Autodesk Inventor part; units mm, degrees
(part 2 of 2)
  arc A137 (24.76, -34.525) -> (24.36, -34.125) centre (24.36, -34.525) ccw
  line L182 (132.16, -34.125) -> (135.12, -34.125)
  arc A138 (135.52, -34.525) -> (135.12, -34.125) centre (135.12, -34.525) ccw
  line L183 (135.52, -34.525) -> (135.52, -47.125)
  arc A139 (132.380606, -52.964154) -> (135.52, -47.125) centre (128.52, -47.125) ccw
  arc A140 (131.76, -52.630488) -> (132.380606, -52.964154) centre (132.16, -52.630488) ccw
  line L184 (131.76, -52.630488) -> (131.76, -34.525)
  arc A141 (132.16, -34.125) -> (131.76, -34.525) centre (132.16, -34.525) ccw
  line L185 (120.76, -34.525) -> (120.76, -53.725)
  arc A142 (120.36, -54.125) -> (120.76, -53.725) centre (120.36, -53.725) ccw
  line L186 (120.36, -54.125) -> (116.16, -54.125)
  arc A143 (115.76, -53.725) -> (116.16, -54.125) centre (116.16, -53.725) ccw
  line L187 (115.76, -53.725) -> (115.76, -34.525)
  arc A144 (116.16, -34.125) -> (115.76, -34.525) centre (116.16, -34.525) ccw
  line L188 (116.16, -34.125) -> (120.36, -34.125)
  arc A145 (120.76, -34.525) -> (120.36, -34.125) centre (120.36, -34.525) ccw
  line L189 (120.36, 2) -> (117.866824, 2)
  arc A146 (117.866824, 2) -> (115.76, 14.782046) centre (65.9053, 0) ccw
  line L190 (115.76, 14.782046) -> (115.76, 29.725)
  arc A147 (116.16, 30.125) -> (115.76, 29.725) centre (116.16, 29.725) ccw
  line L191 (116.16, 30.125) -> (120.36, 30.125)
  arc A148 (120.76, 29.725) -> (120.36, 30.125) centre (120.36, 29.725) ccw
  line L192 (120.76, 29.725) -> (120.76, 2.4)
  arc A149 (120.36, 2) -> (120.76, 2.4) centre (120.36, 2.4) ccw
  line L193 (13.943776, 2) -> (12.16, 2)
  arc A150 (11.76, 2.4) -> (12.16, 2) centre (12.16, 2.4) ccw
  line L194 (11.76, 2.4) -> (11.76, 29.725)
  arc A151 (12.16, 30.125) -> (11.76, 29.725) centre (12.16, 29.725) ccw
  line L195 (12.16, 30.125) -> (16.36, 30.125)
  arc A152 (16.76, 29.725) -> (16.36, 30.125) centre (16.36, 29.725) ccw
  line L196 (16.76, 29.725) -> (16.76, 16.992336)
  arc A153 (16.76, 16.992336) -> (13.943776, 2) centre (65.9053, 0) ccw
  line L197 (135.12, 2) -> (132.16, 2)
  arc A154 (131.76, 2.4) -> (132.16, 2) centre (132.16, 2.4) ccw
  line L198 (131.76, 2.4) -> (131.76, 29.725)
  arc A155 (132.16, 30.125) -> (131.76, 29.725) centre (132.16, 29.725) ccw
  line L199 (132.16, 30.125) -> (135.12, 30.125)
  arc A156 (135.52, 29.725) -> (135.12, 30.125) centre (135.12, 29.725) ccw
  line L200 (135.52, 29.725) -> (135.52, 2.4)
  arc A157 (135.12, 2) -> (135.52, 2.4) centre (135.12, 2.4) ccw
  line L201 (124.16, -2) -> (128.36, -2)
  arc A158 (128.76, -2.4) -> (128.36, -2) centre (128.36, -2.4) ccw
  line L202 (128.76, -2.4) -> (128.76, -29.725)
  arc A159 (128.36, -30.125) -> (128.76, -29.725) centre (128.36, -29.725) ccw
  line L203 (128.36, -30.125) -> (124.16, -30.125)
  arc A160 (123.76, -29.725) -> (124.16, -30.125) centre (124.16, -29.725) ccw
  line L204 (123.76, -29.725) -> (123.76, -2.4)
  arc A161 (124.16, -2) -> (123.76, -2.4) centre (124.16, -2.4) ccw
  line L205 (8.36, 2) -> (5.4, 2)
  arc A162 (5, 2.4) -> (5.4, 2) centre (5.4, 2.4) ccw
  line L206 (5, 2.4) -> (5, 29.725)
  arc A163 (5.4, 30.125) -> (5, 29.725) centre (5.4, 29.725) ccw
  line L207 (5.4, 30.125) -> (8.36, 30.125)
  arc A164 (8.76, 29.725) -> (8.36, 30.125) centre (8.36, 29.725) ccw
  line L208 (8.76, 29.725) -> (8.76, 2.4)
  arc A165 (8.36, 2) -> (8.76, 2.4) centre (8.36, 2.4) ccw
  line L209 (120.76, -2.4) -> (120.76, -29.725)
  arc A166 (120.36, -30.125) -> (120.76, -29.725) centre (120.36, -29.725) ccw
  line L210 (120.36, -30.125) -> (116.16, -30.125)
  arc A167 (115.76, -29.725) -> (116.16, -30.125) centre (116.16, -29.725) ccw
  line L211 (115.76, -29.725) -> (115.76, -14.782046)
  arc A168 (115.76, -14.782046) -> (117.866824, -2) centre (65.9053, 0) ccw
  line L212 (117.866824, -2) -> (120.36, -2)
  arc A169 (120.76, -2.4) -> (120.36, -2) centre (120.36, -2.4) ccw
  line L213 (123.76, 2.4) -> (123.76, 29.725)
  arc A170 (124.16, 30.125) -> (123.76, 29.725) centre (124.16, 29.725) ccw
  line L214 (124.16, 30.125) -> (128.36, 30.125)
  arc A171 (128.76, 29.725) -> (128.36, 30.125) centre (128.36, 29.725) ccw
  line L215 (128.76, 29.725) -> (128.76, 2.4)
  arc A172 (128.36, 2) -> (128.76, 2.4) centre (128.36, 2.4) ccw
  line L216 (128.36, 2) -> (124.16, 2)
  arc A173 (123.76, 2.4) -> (124.16, 2) centre (124.16, 2.4) ccw
  line L217 (135.52, -2.4) -> (135.52, -29.725)
  arc A174 (135.12, -30.125) -> (135.52, -29.725) centre (135.12, -29.725) ccw
  line L218 (135.12, -30.125) -> (132.16, -30.125)
  arc A175 (131.76, -29.725) -> (132.16, -30.125) centre (132.16, -29.725) ccw
  line L219 (131.76, -29.725) -> (131.76, -2.4)
  arc A176 (132.16, -2) -> (131.76, -2.4) centre (132.16, -2.4) ccw
  line L220 (132.16, -2) -> (135.12, -2)
  arc A177 (135.52, -2.4) -> (135.12, -2) centre (135.12, -2.4) ccw
  line L221 (8.76, -2.4) -> (8.76, -29.725)
  arc A178 (8.36, -30.125) -> (8.76, -29.725) centre (8.36, -29.725) ccw
  line L222 (8.36, -30.125) -> (5.4, -30.125)
  arc A179 (5, -29.725) -> (5.4, -30.125) centre (5.4, -29.725) ccw
  line L223 (5, -29.725) -> (5, -2.4)
  arc A180 (5.4, -2) -> (5, -2.4) centre (5.4, -2.4) ccw
  line L224 (5.4, -2) -> (8.36, -2)
  arc A181 (8.76, -2.4) -> (8.36, -2) centre (8.36, -2.4) ccw
  arc A182 (13.943776, -2) -> (16.76, -16.992336) centre (65.9053, 0) ccw
  line L225 (16.76, -16.992336) -> (16.76, -29.725)
  arc A183 (16.36, -30.125) -> (16.76, -29.725) centre (16.36, -29.725) ccw
  line L226 (16.36, -30.125) -> (12.16, -30.125)
  arc A184 (11.76, -29.725) -> (12.16, -30.125) centre (12.16, -29.725) ccw
  line L227 (11.76, -29.725) -> (11.76, -2.4)
  arc A185 (12.16, -2) -> (11.76, -2.4) centre (12.16, -2.4) ccw
  line L228 (12.16, -2) -> (13.943776, -2)
  arc A186 (8.170583, -52.982797) -> (12.16, -54.125) centre (13.033749, -43.53513) ccw
  line L229 (12.16, -34.125) -> (8.36, -34.125)
  line L230 (143.52, -61.875) -> (143.52, 62.125)
  line L231 (143.52, 62.125) -> (-2.75, 62.125)
  point P0 (0, 0)
  point P1 (8.183841, -52.989609)
  point P2 (12.091903, -54.119161)
  constraints: 3 point on circle, 2 end point, 1 centre point, 1 point on line
extrude "Extrusion11" cut sketch "Sketch13" against normal through all contours L17 L229 A34 L33 A33 A186 A17 A18 L19 A19
sketch "Sketch14" plane through (0, 0, 16.5) normal (0, 0, 1) x (1, 0, 0)
  arc A0 (13.943776, -2) -> (16.76, -16.992336) centre (65.9053, 0) ccw
  line L0 (16.76, -16.992336) -> (16.76, -29.725)
  arc A1 (16.36, -30.125) -> (16.76, -29.725) centre (16.36, -29.725) ccw
  line L1 (16.36, -30.125) -> (12.16, -30.125)
  arc A2 (11.76, -29.725) -> (12.16, -30.125) centre (12.16, -29.725) ccw
  line L2 (11.76, -29.725) -> (11.76, -2.4)
  arc A3 (12.16, -2) -> (11.76, -2.4) centre (12.16, -2.4) ccw
  line L3 (12.16, -2) -> (13.943776, -2)
  line L4 (8.76, -2.4) -> (8.76, -29.725)
  arc A4 (8.36, -30.125) -> (8.76, -29.725) centre (8.36, -29.725) ccw
  line L5 (8.36, -30.125) -> (5.4, -30.125)
  arc A5 (5, -29.725) -> (5.4, -30.125) centre (5.4, -29.725) ccw
  line L6 (5, -29.725) -> (5, -2.4)
  arc A6 (5.4, -2) -> (5, -2.4) centre (5.4, -2.4) ccw
  line L7 (5.4, -2) -> (8.36, -2)
  arc A7 (8.76, -2.4) -> (8.36, -2) centre (8.36, -2.4) ccw
  line L8 (135.52, -2.4) -> (135.52, -29.725)
  arc A8 (135.12, -30.125) -> (135.52, -29.725) centre (135.12, -29.725) ccw
  line L9 (135.12, -30.125) -> (132.16, -30.125)
  arc A9 (131.76, -29.725) -> (132.16, -30.125) centre (132.16, -29.725) ccw
  line L10 (131.76, -29.725) -> (131.76, -2.4)
  arc A10 (132.16, -2) -> (131.76, -2.4) centre (132.16, -2.4) ccw
  line L11 (132.16, -2) -> (135.12, -2)
  arc A11 (135.52, -2.4) -> (135.12, -2) centre (135.12, -2.4) ccw
  line L12 (123.76, 2.4) -> (123.76, 29.725)
  arc A12 (124.16, 30.125) -> (123.76, 29.725) centre (124.16, 29.725) ccw
  line L13 (124.16, 30.125) -> (128.36, 30.125)
  arc A13 (128.76, 29.725) -> (128.36, 30.125) centre (128.36, 29.725) ccw
  line L14 (128.76, 29.725) -> (128.76, 2.4)
  arc A14 (128.36, 2) -> (128.76, 2.4) centre (128.36, 2.4) ccw
  line L15 (128.36, 2) -> (124.16, 2)
  arc A15 (123.76, 2.4) -> (124.16, 2) centre (124.16, 2.4) ccw
  line L16 (120.76, -2.4) -> (120.76, -29.725)
  arc A16 (120.36, -30.125) -> (120.76, -29.725) centre (120.36, -29.725) ccw
  line L17 (120.36, -30.125) -> (116.16, -30.125)
  arc A17 (115.76, -29.725) -> (116.16, -30.125) centre (116.16, -29.725) ccw
  line L18 (115.76, -29.725) -> (115.76, -14.782046)
  arc A18 (115.76, -14.782046) -> (117.866824, -2) centre (65.9053, 0) ccw
  line L19 (117.866824, -2) -> (120.36, -2)
  arc A19 (120.76, -2.4) -> (120.36, -2) centre (120.36, -2.4) ccw
  line L20 (8.36, 2) -> (5.4, 2)
  arc A20 (5, 2.4) -> (5.4, 2) centre (5.4, 2.4) ccw
  line L21 (5, 2.4) -> (5, 29.725)
  arc A21 (5.4, 30.125) -> (5, 29.725) centre (5.4, 29.725) ccw
  line L22 (5.4, 30.125) -> (8.36, 30.125)
  arc A22 (8.76, 29.725) -> (8.36, 30.125) centre (8.36, 29.725) ccw
  line L23 (8.76, 29.725) -> (8.76, 2.4)
  arc A23 (8.36, 2) -> (8.76, 2.4) centre (8.36, 2.4) ccw
  line L24 (124.16, -2) -> (128.36, -2)
  arc A24 (128.76, -2.4) -> (128.36, -2) centre (128.36, -2.4) ccw
  line L25 (128.76, -2.4) -> (128.76, -29.725)
  arc A25 (128.36, -30.125) -> (128.76, -29.725) centre (128.36, -29.725) ccw
  line L26 (128.36, -30.125) -> (124.16, -30.125)
  arc A26 (123.76, -29.725) -> (124.16, -30.125) centre (124.16, -29.725) ccw
  line L27 (123.76, -29.725) -> (123.76, -2.4)
  arc A27 (124.16, -2) -> (123.76, -2.4) centre (124.16, -2.4) ccw
  line L28 (135.12, 2) -> (132.16, 2)
  arc A28 (131.76, 2.4) -> (132.16, 2) centre (132.16, 2.4) ccw
  line L29 (131.76, 2.4) -> (131.76, 29.725)
  arc A29 (132.16, 30.125) -> (131.76, 29.725) centre (132.16, 29.725) ccw
  line L30 (132.16, 30.125) -> (135.12, 30.125)
  arc A30 (135.52, 29.725) -> (135.12, 30.125) centre (135.12, 29.725) ccw
  line L31 (135.52, 29.725) -> (135.52, 2.4)
  arc A31 (135.12, 2) -> (135.52, 2.4) centre (135.12, 2.4) ccw
  line L32 (13.943776, 2) -> (12.16, 2)
  arc A32 (11.76, 2.4) -> (12.16, 2) centre (12.16, 2.4) ccw
  line L33 (11.76, 2.4) -> (11.76, 29.725)
  arc A33 (12.16, 30.125) -> (11.76, 29.725) centre (12.16, 29.725) ccw
  line L34 (12.16, 30.125) -> (16.36, 30.125)
  arc A34 (16.76, 29.725) -> (16.36, 30.125) centre (16.36, 29.725) ccw
  line L35 (16.76, 29.725) -> (16.76, 16.992336)
  arc A35 (16.76, 16.992336) -> (13.943776, 2) centre (65.9053, 0) ccw
  line L36 (120.36, 2) -> (117.866824, 2)
  arc A36 (117.866824, 2) -> (115.76, 14.782046) centre (65.9053, 0) ccw
  line L37 (115.76, 14.782046) -> (115.76, 29.725)
  arc A37 (116.16, 30.125) -> (115.76, 29.725) centre (116.16, 29.725) ccw
  line L38 (116.16, 30.125) -> (120.36, 30.125)
  arc A38 (120.76, 29.725) -> (120.36, 30.125) centre (120.36, 29.725) ccw
  line L39 (120.76, 29.725) -> (120.76, 2.4)
  arc A39 (120.36, 2) -> (120.76, 2.4) centre (120.36, 2.4) ccw
  line L40 (120.76, -34.525) -> (120.76, -53.725)
  arc A40 (120.36, -54.125) -> (120.76, -53.725) centre (120.36, -53.725) ccw
  line L41 (120.36, -54.125) -> (116.16, -54.125)
  arc A41 (115.76, -53.725) -> (116.16, -54.125) centre (116.16, -53.725) ccw
  line L42 (115.76, -53.725) -> (115.76, -34.525)
  arc A42 (116.16, -34.125) -> (115.76, -34.525) centre (116.16, -34.525) ccw
  line L43 (116.16, -34.125) -> (120.36, -34.125)
  arc A43 (120.76, -34.525) -> (120.36, -34.125) centre (120.36, -34.525) ccw
  line L44 (132.16, -34.125) -> (135.12, -34.125)
  arc A44 (135.52, -34.525) -> (135.12, -34.125) centre (135.12, -34.525) ccw
  line L45 (135.52, -34.525) -> (135.52, -47.125)
  arc A45 (132.380606, -52.964154) -> (135.52, -47.125) centre (128.52, -47.125) ccw
  arc A46 (131.76, -52.630488) -> (132.380606, -52.964154) centre (132.16, -52.630488) ccw
  line L46 (131.76, -52.630488) -> (131.76, -34.525)
  arc A47 (132.16, -34.125) -> (131.76, -34.525) centre (132.16, -34.525) ccw
  line L47 (24.76, -34.525) -> (24.76, -53.725)
  arc A48 (24.36, -54.125) -> (24.76, -53.725) centre (24.36, -53.725) ccw
  line L48 (24.36, -54.125) -> (20.16, -54.125)
  arc A49 (19.76, -53.725) -> (20.16, -54.125) centre (20.16, -53.725) ccw
  line L49 (19.76, -53.725) -> (19.76, -34.525)
  arc A50 (20.16, -34.125) -> (19.76, -34.525) centre (20.16, -34.525) ccw
  line L50 (20.16, -34.125) -> (24.36, -34.125)
  arc A51 (24.76, -34.525) -> (24.36, -34.125) centre (24.36, -34.525) ccw
  arc A52 (23.520345, 30.125) -> (19.76, 23.971051) centre (65.9053, 0) ccw
  line L51 (19.76, 23.971051) -> (19.76, 29.725)
  arc A53 (20.16, 30.125) -> (19.76, 29.725) centre (20.16, 29.725) ccw
  line L52 (20.16, 30.125) -> (23.520345, 30.125)
  line L53 (107.76, 34.525) -> (107.76, 53.725)
  arc A54 (108.16, 54.125) -> (107.76, 53.725) centre (108.16, 53.725) ccw
  line L54 (108.16, 54.125) -> (112.36, 54.125)
  arc A55 (112.76, 53.725) -> (112.36, 54.125) centre (112.36, 53.725) ccw
  line L55 (112.76, 53.725) -> (112.76, 34.525)
  arc A56 (112.36, 34.125) -> (112.76, 34.525) centre (112.36, 34.525) ccw
  line L56 (112.36, 34.125) -> (108.16, 34.125)
  arc A57 (107.76, 34.525) -> (108.16, 34.125) centre (108.16, 34.525) ccw
  arc A58 (108.290254, -30.125) -> (112.76, -22.552984) centre (65.9053, 0) ccw
  line L57 (112.76, -22.552984) -> (112.76, -29.725)
  arc A59 (112.36, -30.125) -> (112.76, -29.725) centre (112.36, -29.725) ccw
  line L58 (112.36, -30.125) -> (108.290254, -30.125)
  line L59 (128.76, -34.525) -> (128.76, -53.725)
  arc A60 (128.36, -54.125) -> (128.76, -53.725) centre (128.36, -53.725) ccw
  line L60 (128.36, -54.125) -> (124.16, -54.125)
  arc A61 (123.76, -53.725) -> (124.16, -54.125) centre (124.16, -53.725) ccw
  line L61 (123.76, -53.725) -> (123.76, -34.525)
  arc A62 (124.16, -34.125) -> (123.76, -34.525) centre (124.16, -34.525) ccw
  line L62 (124.16, -34.125) -> (128.36, -34.125)
  arc A63 (128.76, -34.525) -> (128.36, -34.125) centre (128.36, -34.525) ccw
  line L63 (16.36, 34.125) -> (12.16, 34.125)
  arc A64 (11.76, 34.525) -> (12.16, 34.125) centre (12.16, 34.525) ccw
  line L64 (11.76, 34.525) -> (11.76, 53.725)
  arc A65 (12.16, 54.125) -> (11.76, 53.725) centre (12.16, 53.725) ccw
  line L65 (12.16, 54.125) -> (16.36, 54.125)
  arc A66 (16.76, 53.725) -> (16.36, 54.125) centre (16.36, 53.725) ccw
  line L66 (16.76, 53.725) -> (16.76, 34.525)
  arc A67 (16.36, 34.125) -> (16.76, 34.525) centre (16.36, 34.525) ccw
  line L67 (8.36, 34.125) -> (5.4, 34.125)
  arc A68 (5, 34.525) -> (5.4, 34.125) centre (5.4, 34.525) ccw
  line L68 (5, 34.525) -> (5, 47.125)
  arc A69 (8.139394, 52.964154) -> (5, 47.125) centre (12, 47.125) ccw
  arc A70 (8.76, 52.630488) -> (8.139394, 52.964154) centre (8.36, 52.630488) ccw
  line L69 (8.76, 52.630488) -> (8.76, 34.525)
  arc A71 (8.36, 34.125) -> (8.76, 34.525) centre (8.36, 34.525) ccw
  line L70 (115.76, 34.525) -> (115.76, 53.725)
  arc A72 (116.16, 54.125) -> (115.76, 53.725) centre (116.16, 53.725) ccw
  line L71 (116.16, 54.125) -> (120.36, 54.125)
  arc A73 (120.76, 53.725) -> (120.36, 54.125) centre (120.36, 53.725) ccw
  line L72 (120.76, 53.725) -> (120.76, 34.525)
  arc A74 (120.36, 34.125) -> (120.76, 34.525) centre (120.36, 34.525) ccw
  line L73 (120.36, 34.125) -> (116.16, 34.125)
  arc A75 (115.76, 34.525) -> (116.16, 34.125) centre (116.16, 34.525) ccw
  line L74 (83.76, -12.185449) -> (83.76, 0.332706)
  line L75 (83.76, 0.332706) -> (88.76, 13.193084)
  line L76 (88.76, 13.193084) -> (88.76, -9.998135)
  line L77 (88.76, -9.998135) -> (83.76, -12.185449)
  line L78 (80.76, -21.138342) -> (80.76, -42.477499)
  arc A76 (75.76, -43.907686) -> (80.76, -42.477499) centre (65.9053, 0) ccw
  line L79 (75.76, -43.907686) -> (75.76, -23.325656)
  line L80 (75.76, -23.325656) -> (80.76, -21.138342)
  line L81 (91.76, -8.685747) -> (91.76, 20.90931)
  line L82 (91.76, 20.90931) -> (96.47099, 33.026332)
  arc A77 (96.76, 32.756488) -> (96.47099, 33.026332) centre (65.9053, 0) ccw
  line L83 (96.76, 32.756488) -> (96.76, -6.498433)
  line L84 (96.76, -6.498433) -> (91.76, -8.685747)
  line L85 (107.76, -1.686342) -> (107.76, 16.528281)
  arc A78 (110.904226, -0.31086) -> (107.76, 16.528281) centre (65.9053, 0) ccw
  line L86 (110.904226, -0.31086) -> (107.76, -1.686342)
  line L87 (104.76, -10.639235) -> (104.76, -22.700491)
  arc A79 (99.76, -29.645561) -> (104.76, -22.700491) centre (65.9053, 0) ccw
  line L88 (99.76, -29.645561) -> (99.76, -12.826549)
  line L89 (99.76, -12.826549) -> (104.76, -10.639235)
  line L90 (75.76, -0.926469) -> (75.76, 24.326911)
  line L91 (75.76, 24.326911) -> (80.76, 20.268157)
  line L92 (80.76, 20.268157) -> (80.76, 11.933908)
  line L93 (80.76, 11.933908) -> (75.76, -0.926469)
  line L94 (72.76, -27.960124) -> (72.76, -44.474859)
  arc A80 (67.76, -44.961763) -> (72.76, -44.474859) centre (65.9053, 0) ccw
  line L95 (67.76, -44.961763) -> (67.76, -40.820501)
  line L96 (67.76, -40.820501) -> (72.76, -27.960124)
  line L97 (24.76, 34.125) -> (20.16, 34.125)
  arc A81 (19.76, 34.525) -> (20.16, 34.125) centre (20.16, 34.525) ccw
  line L98 (19.76, 34.525) -> (19.76, 53.725)
  arc A82 (20.16, 54.125) -> (19.76, 53.725) centre (20.16, 53.725) ccw
  line L99 (20.16, 54.125) -> (24.36, 54.125)
  arc A83 (24.76, 53.725) -> (24.36, 54.125) centre (24.36, 53.725) ccw
  line L100 (24.76, 53.725) -> (24.76, 34.125)
  line L101 (51.76, -42.718971) -> (51.76, 42.718971)
  arc A84 (52.72419, 43.026252) -> (51.76, 42.718971) centre (65.9053, 0) ccw
  line L102 (52.72419, 43.026252) -> (56.76, 39.750179)
  line L103 (56.76, 39.750179) -> (56.76, -44.060907)
  arc A85 (51.76, -42.718971) -> (56.76, -44.060907) centre (65.9053, 0) ccw
  line L104 (48.76, -49.092145) -> (48.76, -53.725)
  arc A86 (48.36, -54.125) -> (48.76, -53.725) centre (48.36, -53.725) ccw
  line L105 (48.36, -54.125) -> (44.16, -54.125)
  arc A87 (43.76, -53.725) -> (44.16, -54.125) centre (44.16, -53.725) ccw
  line L106 (43.76, -53.725) -> (43.76, -47.048759)
  arc A88 (43.76, -47.048759) -> (48.76, -49.092145) centre (65.9053, 0) ccw
  line L107 (51.76, 50.03909) -> (51.76, 53.725)
  arc A89 (52.16, 54.125) -> (51.76, 53.725) centre (52.16, 53.725) ccw
  line L108 (52.16, 54.125) -> (56.36, 54.125)
  arc A90 (56.76, 53.725) -> (56.36, 54.125) centre (56.36, 53.725) ccw
  line L109 (56.76, 53.725) -> (56.76, 51.189486)
  arc A91 (56.76, 51.189486) -> (51.76, 50.03909) centre (65.9053, 0) ccw
  arc A92 (43.76, -39.173788) -> (48.76, -41.605753) centre (65.9053, 0) ccw
  line L110 (43.76, -39.173788) -> (43.76, 39.173788)
  arc A93 (48.76, 41.605753) -> (43.76, 39.173788) centre (65.9053, 0) ccw
  line L111 (48.76, 41.605753) -> (48.76, -41.605753)
  line L112 (108.16, -34.125) -> (112.36, -34.125)
  arc A94 (112.76, -34.525) -> (112.36, -34.125) centre (112.36, -34.525) ccw
  line L113 (112.76, -34.525) -> (112.76, -53.725)
  arc A95 (112.36, -54.125) -> (112.76, -53.725) centre (112.36, -53.725) ccw
  line L114 (112.36, -54.125) -> (108.16, -54.125)
  arc A96 (107.76, -53.725) -> (108.16, -54.125) centre (108.16, -53.725) ccw
  line L115 (107.76, -53.725) -> (107.76, -34.525)
  arc A97 (108.16, -34.125) -> (107.76, -34.525) centre (108.16, -34.525) ccw
  line L116 (59.76, -42.079676) -> (59.76, 37.314927)
  line L117 (59.76, 37.314927) -> (64.76, 33.256172)
  line L118 (64.76, 33.256172) -> (64.76, -29.219299)
  line L119 (64.76, -29.219299) -> (59.76, -42.079676)
  line L120 (23.520345, -30.125) -> (20.16, -30.125)
  arc A98 (19.76, -29.725) -> (20.16, -30.125) centre (20.16, -29.725) ccw
  line L121 (19.76, -29.725) -> (19.76, -23.971051)
  arc A99 (19.76, -23.971051) -> (23.520345, -30.125) centre (65.9053, 0) ccw
  line L122 (27.76, -23.873334) -> (27.76, 23.873334)
  arc A100 (32.76, 30.436641) -> (27.76, 23.873334) centre (65.9053, 0) ccw
  line L123 (32.76, 30.436641) -> (32.76, -30.436641)
  arc A101 (27.76, -23.873334) -> (32.76, -30.436641) centre (65.9053, 0) ccw
  line L124 (27.76, 35.34029) -> (27.76, 53.725)
  arc A102 (28.16, 54.125) -> (27.76, 53.725) centre (28.16, 53.725) ccw
  line L125 (28.16, 54.125) -> (32.36, 54.125)
  arc A103 (32.76, 53.725) -> (32.36, 54.125) centre (32.36, 53.725) ccw
  line L126 (32.76, 53.725) -> (32.76, 40.067307)
  arc A104 (32.76, 40.067307) -> (27.76, 35.34029) centre (65.9053, 0) ccw
  line L127 (35.76, -33.410491) -> (35.76, 33.410491)
  arc A105 (40.76, 37.319082) -> (35.76, 33.410491) centre (65.9053, 0) ccw
  line L128 (40.76, 37.319082) -> (40.76, -37.319082)
  arc A106 (35.76, -33.410491) -> (40.76, -37.319082) centre (65.9053, 0) ccw
  line L129 (35.76, 42.370519) -> (35.76, 53.725)
  arc A107 (36.16, 54.125) -> (35.76, 53.725) centre (36.16, 53.725) ccw
  line L130 (36.16, 54.125) -> (40.36, 54.125)
  arc A108 (40.76, 53.725) -> (40.36, 54.125) centre (40.36, 53.725) ccw
  line L131 (40.76, 53.725) -> (40.76, 45.516084)
  arc A109 (40.76, 45.516084) -> (35.76, 42.370519) centre (65.9053, 0) ccw
  line L132 (83.76, -19.825953) -> (88.76, -17.63864)
  line L133 (88.76, -17.63864) -> (88.76, -38.764193)
  arc A110 (83.76, -41.306291) -> (88.76, -38.764193) centre (65.9053, 0) ccw
  line L134 (83.76, -41.306291) -> (83.76, -19.825953)
  line L135 (80.76, -49.8331) -> (80.76, -53.725)
  arc A111 (80.36, -54.125) -> (80.76, -53.725) centre (80.36, -53.725) ccw
  line L136 (80.36, -54.125) -> (76.16, -54.125)
  arc A112 (75.76, -53.725) -> (76.16, -54.125) centre (76.16, -53.725) ccw
  line L137 (75.76, -53.725) -> (75.76, -51.057662)
  arc A113 (75.76, -51.057662) -> (80.76, -49.8331) centre (65.9053, 0) ccw
  line L138 (91.76, -16.326251) -> (96.76, -14.138937)
  line L139 (96.76, -14.138937) -> (96.76, -32.756488)
  arc A114 (91.76, -36.831162) -> (96.76, -32.756488) centre (65.9053, 0) ccw
  line L140 (91.76, -36.831162) -> (91.76, -16.326251)
  line L141 (72.76, -51.546223) -> (72.76, -53.725)
  arc A115 (72.36, -54.125) -> (72.76, -53.725) centre (72.36, -53.725) ccw
  line L142 (72.36, -54.125) -> (68.16, -54.125)
  arc A116 (67.76, -53.725) -> (68.16, -54.125) centre (68.16, -53.725) ccw
  line L143 (67.76, -53.725) -> (67.76, -51.966913)
  arc A117 (67.76, -51.966913) -> (72.76, -51.546223) centre (65.9053, 0) ccw
  line L144 (107.76, -9.326846) -> (110.135552, -8.287631)
  arc A118 (107.76, -16.528281) -> (110.135552, -8.287631) centre (65.9053, 0) ccw
  line L145 (107.76, -16.528281) -> (107.76, -9.326846)
  line L146 (104.76, -34.558823) -> (104.76, -53.725)
  arc A119 (104.36, -54.125) -> (104.76, -53.725) centre (104.36, -53.725) ccw
  line L147 (104.36, -54.125) -> (100.16, -54.125)
  arc A120 (99.76, -53.725) -> (100.16, -54.125) centre (100.16, -53.725) ccw
  line L148 (99.76, -53.725) -> (99.76, -39.469726)
  arc A121 (99.76, -39.469726) -> (104.76, -34.558823) centre (65.9053, 0) ccw
  line L149 (91.76, 45.116898) -> (91.76, 53.725)
  arc A122 (92.16, 54.125) -> (91.76, 53.725) centre (92.16, 53.725) ccw
  line L150 (92.16, 54.125) -> (96.36, 54.125)
  arc A123 (96.76, 53.725) -> (96.36, 54.125) centre (96.36, 53.725) ccw
  line L151 (96.76, 53.725) -> (96.76, 41.85675)
  arc A124 (96.76, 41.85675) -> (91.76, 45.116898) centre (65.9053, 0) ccw
  arc A125 (83.76, -48.838609) -> (88.76, -46.708272) centre (65.9053, 0) ccw
  line L152 (88.76, -46.708272) -> (88.76, -53.725)
  arc A126 (88.36, -54.125) -> (88.76, -53.725) centre (88.36, -53.725) ccw
  line L153 (88.36, -54.125) -> (84.16, -54.125)
  arc A127 (83.76, -53.725) -> (84.16, -54.125) centre (84.16, -53.725) ccw
  line L154 (83.76, -53.725) -> (83.76, -48.838609)
  line L155 (88.76, 32.510512) -> (85.887401, 25.121972)
  line L156 (85.887401, 25.121972) -> (83.76, 26.848892)
  line L157 (83.76, 26.848892) -> (83.76, 41.306291)
  arc A128 (88.76, 38.764193) -> (83.76, 41.306291) centre (65.9053, 0) ccw
  line L158 (88.76, 38.764193) -> (88.76, 32.510512)
  line L159 (80.76, 42.477499) -> (80.76, 29.284145)
  line L160 (80.76, 29.284145) -> (75.76, 33.342899)
  line L161 (75.76, 33.342899) -> (75.76, 43.907686)
  arc A129 (80.76, 42.477499) -> (75.76, 43.907686) centre (65.9053, 0) ccw
  line L162 (72.76, 44.474859) -> (72.76, 35.778152)
  line L163 (72.76, 35.778152) -> (67.76, 39.836907)
  line L164 (67.76, 39.836907) -> (67.76, 44.961763)
  arc A130 (72.76, 44.474859) -> (67.76, 44.961763) centre (65.9053, 0) ccw
  line L165 (64.76, 44.985423) -> (64.76, 42.27216)
  line L166 (64.76, 42.27216) -> (61.648183, 44.79818)
  arc A131 (64.76, 44.985423) -> (61.648183, 44.79818) centre (65.9053, 0) ccw
  line L167 (104.76, -2.99873) -> (99.76, -5.186044)
  line L168 (99.76, -5.186044) -> (99.76, 29.645561)
  arc A132 (104.76, 22.700491) -> (99.76, 29.645561) centre (65.9053, 0) ccw
  line L169 (104.76, 22.700491) -> (104.76, -2.99873)
  line L170 (80.76, -13.497837) -> (77.895632, -14.750892)
  line L171 (77.895632, -14.750892) -> (80.76, -7.38352)
  line L172 (80.76, -7.38352) -> (80.76, -13.497837)
  arc A133 (64.76, 51.987386) -> (59.76, 51.635601) centre (65.9053, 0) ccw
  line L173 (59.76, 51.635601) -> (59.76, 53.725)
  arc A134 (60.16, 54.125) -> (59.76, 53.725) centre (60.16, 53.725) ccw
  line L174 (60.16, 54.125) -> (64.36, 54.125)
  arc A135 (64.76, 53.725) -> (64.36, 54.125) centre (64.36, 53.725) ccw
  line L175 (64.76, 53.725) -> (64.76, 51.987386)
  line L176 (72.76, -8.642695) -> (67.76, -21.503073)
  line L177 (67.76, -21.503073) -> (67.76, 30.820919)
  line L178 (67.76, 30.820919) -> (72.76, 26.762164)
  line L179 (72.76, 26.762164) -> (72.76, -8.642695)
  arc A136 (80.76, 49.8331) -> (75.76, 51.057662) centre (65.9053, 0) ccw
  line L180 (75.76, 51.057662) -> (75.76, 53.725)
  arc A137 (76.16, 54.125) -> (75.76, 53.725) centre (76.16, 53.725) ccw
  line L181 (76.16, 54.125) -> (80.36, 54.125)
  arc A138 (80.76, 53.725) -> (80.36, 54.125) centre (80.36, 53.725) ccw
  line L182 (80.76, 53.725) -> (80.76, 49.8331)
  arc A139 (88.76, 46.708272) -> (83.76, 48.838609) centre (65.9053, 0) ccw
  line L183 (83.76, 48.838609) -> (83.76, 53.725)
  arc A140 (84.16, 54.125) -> (83.76, 53.725) centre (84.16, 53.725) ccw
  line L184 (84.16, 54.125) -> (88.36, 54.125)
  arc A141 (88.76, 53.725) -> (88.36, 54.125) centre (88.36, 53.725) ccw
  line L185 (88.76, 53.725) -> (88.76, 46.708272)
  arc A142 (104.76, 34.558823) -> (99.76, 39.469726) centre (65.9053, 0) ccw
  line L186 (99.76, 39.469726) -> (99.76, 53.725)
  arc A143 (100.16, 54.125) -> (99.76, 53.725) centre (100.16, 53.725) ccw
  line L187 (100.16, 54.125) -> (104.36, 54.125)
  arc A144 (104.76, 53.725) -> (104.36, 54.125) centre (104.36, 53.725) ccw
  line L188 (104.76, 53.725) -> (104.76, 34.558823)
  arc A145 (91.76, -45.116898) -> (96.76, -41.85675) centre (65.9053, 0) ccw
  line L189 (96.76, -41.85675) -> (96.76, -53.725)
  arc A146 (96.36, -54.125) -> (96.76, -53.725) centre (96.36, -53.725) ccw
  line L190 (96.36, -54.125) -> (92.16, -54.125)
  arc A147 (91.76, -53.725) -> (92.16, -54.125) centre (92.16, -53.725) ccw
  line L191 (91.76, -53.725) -> (91.76, -45.116898)
  arc A148 (72.76, 51.546223) -> (67.76, 51.966913) centre (65.9053, 0) ccw
  line L192 (67.76, 51.966913) -> (67.76, 53.725)
  arc A149 (68.16, 54.125) -> (67.76, 53.725) centre (68.16, 53.725) ccw
  line L193 (68.16, 54.125) -> (72.36, 54.125)
  arc A150 (72.76, 53.725) -> (72.36, 54.125) centre (72.36, 53.725) ccw
  line L194 (72.76, 53.725) -> (72.76, 51.546223)
  line L195 (5.4, -34.125) -> (16.36, -34.125)
  arc A151 (16.76, -34.525) -> (16.36, -34.125) centre (16.36, -34.525) ccw
  line L196 (16.76, -34.525) -> (16.76, -53.725)
  arc A152 (16.36, -54.125) -> (16.76, -53.725) centre (16.36, -53.725) ccw
  line L197 (16.36, -54.125) -> (12.16, -54.125)
  arc A153 (12.091903, -54.119161) -> (12.16, -54.125) centre (12.16, -53.725) ccw
  arc A154 (8.183841, -52.989609) -> (12.091903, -54.119161) centre (13.033749, -43.53513) ccw
  arc A155 (8.139394, -52.964154) -> (8.183841, -52.989609) centre (8.36, -52.630488) ccw
  arc A156 (5, -47.125) -> (8.139394, -52.964154) centre (12, -47.125) ccw
  line L198 (5, -47.125) -> (5, -34.525)
  arc A157 (5.4, -34.125) -> (5, -34.525) centre (5.4, -34.525) ccw
  arc A158 (51.76, -50.03909) -> (56.76, -51.189486) centre (65.9053, 0) ccw
  line L199 (56.76, -51.189486) -> (56.76, -53.725)
  arc A159 (56.36, -54.125) -> (56.76, -53.725) centre (56.36, -53.725) ccw
  line L200 (56.36, -54.125) -> (52.16, -54.125)
  arc A160 (51.76, -53.725) -> (52.16, -54.125) centre (52.16, -53.725) ccw
  line L201 (51.76, -53.725) -> (51.76, -50.03909)
  arc A161 (24.76, 18.222631) -> (24.76, -18.222631) centre (65.9053, 0) ccw
  line L202 (24.76, 18.222631) -> (24.76, -18.222631)
  arc A162 (35.76, -42.370519) -> (40.76, -45.516084) centre (65.9053, 0) ccw
  line L203 (40.76, -45.516084) -> (40.76, -53.725)
  arc A163 (40.36, -54.125) -> (40.76, -53.725) centre (40.36, -53.725) ccw
  line L204 (40.36, -54.125) -> (36.16, -54.125)
  arc A164 (35.76, -53.725) -> (36.16, -54.125) centre (36.16, -53.725) ccw
  line L205 (35.76, -53.725) -> (35.76, -42.370519)
  line L206 (135.12, 34.125) -> (132.16, 34.125)
  arc A165 (131.76, 34.525) -> (132.16, 34.125) centre (132.16, 34.525) ccw
  line L207 (131.76, 34.525) -> (131.76, 52.630488)
  arc A166 (132.380606, 52.964154) -> (131.76, 52.630488) centre (132.16, 52.630488) ccw
  arc A167 (135.52, 47.125) -> (132.380606, 52.964154) centre (128.52, 47.125) ccw
  line L208 (135.52, 47.125) -> (135.52, 34.525)
  arc A168 (135.12, 34.125) -> (135.52, 34.525) centre (135.12, 34.525) ccw
  line L209 (128.36, 34.125) -> (124.16, 34.125)
  arc A169 (123.76, 34.525) -> (124.16, 34.125) centre (124.16, 34.525) ccw
  line L210 (123.76, 34.525) -> (123.76, 53.725)
  arc A170 (124.16, 54.125) -> (123.76, 53.725) centre (124.16, 53.725) ccw
  line L211 (124.16, 54.125) -> (128.36, 54.125)
  arc A171 (128.76, 53.725) -> (128.36, 54.125) centre (128.36, 53.725) ccw
  line L212 (128.76, 53.725) -> (128.76, 34.525)
  arc A172 (128.36, 34.125) -> (128.76, 34.525) centre (128.36, 34.525) ccw
  arc A173 (27.76, -35.34029) -> (32.76, -40.067307) centre (65.9053, 0) ccw
  line L213 (32.76, -40.067307) -> (32.76, -53.725)
  arc A174 (32.36, -54.125) -> (32.76, -53.725) centre (32.36, -53.725) ccw
  line L214 (32.36, -54.125) -> (28.16, -54.125)
  arc A175 (27.76, -53.725) -> (28.16, -54.125) centre (28.16, -53.725) ccw
  line L215 (27.76, -53.725) -> (27.76, -35.34029)
  arc A176 (59.76, -51.635601) -> (64.76, -51.987386) centre (65.9053, 0) ccw
  line L216 (64.76, -51.987386) -> (64.76, -53.725)
  arc A177 (64.36, -54.125) -> (64.76, -53.725) centre (64.36, -53.725) ccw
  line L217 (64.36, -54.125) -> (60.16, -54.125)
  arc A178 (59.76, -53.725) -> (60.16, -54.125) centre (60.16, -53.725) ccw
  line L218 (59.76, -53.725) -> (59.76, -51.635601)
  line L219 (108.290254, 30.125) -> (112.36, 30.125)
  arc A179 (112.76, 29.725) -> (112.36, 30.125) centre (112.36, 29.725) ccw
  line L220 (112.76, 29.725) -> (112.76, 22.552984)
  arc A180 (112.76, 22.552984) -> (108.290254, 30.125) centre (65.9053, 0) ccw
  arc A181 (48.76, 49.092145) -> (43.76, 47.048759) centre (65.9053, 0) ccw
  line L221 (43.76, 47.048759) -> (43.76, 53.725)
  arc A182 (44.16, 54.125) -> (43.76, 53.725) centre (44.16, 53.725) ccw
  line L222 (44.16, 54.125) -> (48.36, 54.125)
  arc A183 (48.76, 53.725) -> (48.36, 54.125) centre (48.36, 53.725) ccw
  line L223 (48.76, 53.725) -> (48.76, 49.092145)
  line L224 (143.52, -61.875) -> (7, -61.875)
  line L225 (-2.75, -52.125) -> (-2.75, 62.125)
  arc A184 (-2.75, -52.125) -> (7, -61.875) centre (7, -52.125) ccw
  arc A185 (19.76, -53.725) -> (20.16, -54.125) centre (20.16, -53.725) ccw
  arc A186 (16.76, -34.525) -> (16.36, -34.125) centre (16.36, -34.525) ccw
  line L226 (19.76, -53.725) -> (16.76, -53.725)
  line L227 (16.76, -53.725) -> (16.76, -34.525)
  line L228 (16.76, -34.525) -> (19.76, -34.525)
  line L229 (19.76, -34.525) -> (19.76, -53.725)
  line L230 (24.76, -53.725) -> (24.76, -34.525)
  line L231 (24.76, -50.125) -> (19.76, -50.125)
  line L232 (19.76, -50.125) -> (19.76, -47.125)
  line L233 (19.76, -47.125) -> (24.76, -47.125)
  line L234 (24.76, -47.125) -> (24.76, -50.125)
  line L235 (19.76, -44.125) -> (24.76, -44.125)
  line L236 (24.76, -38.125) -> (19.76, -38.125)
  line L237 (19.76, -41.125) -> (24.76, -41.125)
  line L238 (143.52, -61.875) -> (143.52, 62.125)
  line L239 (143.52, 62.125) -> (-2.75, 62.125)
  point P0 (0, 0)
  dimension "d105" = 3
  dimension "d106" = 3
  constraints: 22 end point, 4 parallel, 4 symmetric about line, 2 horizontal, 2 midpoint, 2 perpendicular, 2 point on line
  measures "d105" distance of L231.end L232.end
  measures "d106" distance between parallel lines of L235 L233
extrude "Extrusion12" add sketch "Sketch14" against normal up to surface (1.5 mm away) contours L47 L237 L49 L236 | L47 L231 L49 L233
sketch "Sketch15" plane through (0, 0, 0) normal (0, 0, -1) x (-1, 0, 0)
  line L0 (-143.52, -62.125) -> (-143.52, 62.125) projected
  line L1 (-7, -62.125) -> (-143.52, -62.125) projected
  arc A0 (-7, -62.125) -> (3, -52.125) centre (-7, -52.125) ccw projected
  line L2 (3, 62.125) -> (3, -52.125) projected
  line L3 (-143.52, 62.125) -> (3, 62.125) projected
  line L4 (-3, -51.125) -> (-3, 56.125) projected
  arc A1 (-8, -56.125) -> (-3, -51.125) centre (-8, -51.125) ccw projected
  line L5 (-137.52, -56.125) -> (-8, -56.125) projected
  line L6 (-137.52, 56.125) -> (-137.52, -56.125) projected
  line L7 (-3, 56.125) -> (-137.52, 56.125) projected
  line L8 (-140.52, 59.125) -> (-140.52, -59.125)
  line L9 (-140.52, -59.125) -> (-8, -59.125)
  arc A2 (-8, -59.125) -> (0, -51.125) centre (-8, -51.125) ccw
  line L10 (0, -51.125) -> (0, 59.125)
  line L11 (0, 59.125) -> (-140.52, 59.125)
  point P0 (0, 0)
  dimension "d109" = 3
  constraints: 8 end point, 2 point on circle, 1 centre point, 4 other
  measures "d109" distance between parallel lines of L7 L11
extrude "Extrusion13" cut sketch "Sketch15" against normal blind 5 contours A1 L5 L6 L7 L4 | L11 L10 A2 L9 L8
sketch "Sketch16" plane through (7, -62.125, 0) normal (0, -1, 0) x (1, 0, 0)
  line L0 (136.52, 0) -> (136.52, 16.25) projected
  line L1 (0, 0) -> (136.52, 0) projected
  circle A0 centre (121.52, 0) radius 4
  point P0 (-7, 0)
  point P1 (125.52, 0)
  point P2 (117.52, 0)
  dimension "d112" = 15
  dimension "d113" = 0
  dimension "d114" = 8
  constraints: 1 centre point, 1 coincident
  measures "d112" distance from line of L0 point (121.52, 0)
  measures "d113" distance from line of point (121.52, 0) L1
  measures "d114" diameter of A0
extrude "Extrusion14" add sketch "Sketch16" against normal up to surface (3 mm away) contours L1 A0 picked at (121.359284, -1.323612)
sketch "Sketch17" plane through (7, -62.125, 16.25) normal (0, -1, 0) x (1, 0, 0)
  arc A0 (117.52, -16.25) -> (125.52, -16.25) centre (121.52, -16.25) ccw projected
  point P0 (-7, -16.25)
  constraints: 1 coincident
hole "Hole2" at (128.52, -62.125, 0) direction (0, 1, 0) diameter 3.4 depth 8 clearance for "Socket Head Cap Screw" size "M3" standard "Ansi Metric M Profile"
fillet "Fillet7" radius 1 2 edges at (124.52, -60.625, 0) (132.52, -60.625, 0)
sketch "Sketch18" plane through (-3, -52.125, 0) normal (-1, 0, 0) x (0, 0, 1)
  line L0 (0, 114.25) -> (16.25, 114.25) projected
  circle A0 centre (0, 34.25) radius 4
  point P0 (0, 52.125)
  dimension "d125" = 80
  dimension "d126" = 8
  constraints: 1 centre point, 1 coincident
  measures "d125" distance from line of point (0, 34.25) L0
  measures "d126" diameter of A0
extrude "Extrusion15" add sketch "Sketch18" against normal up to surface (3 mm away)
fillet "Fillet8" radius 1 2 edges at (-1.5, -13.875, 0) (-1.5, -21.875, 0)
sketch "Sketch19" plane through (-3, -52.125, 16.25) normal (-1, 0, 0) x (0, 0, 1)
  arc A0 (-17.05, 38.169184) -> (-17.05, 30.330816) centre (-16.25, 34.25) ccw
  point P0 (-16.25, 52.125)
hole "Hole3" at (-3, -17.875, 0) direction (1, 0, 0) diameter 3.4 depth 8 clearance for "Socket Head Cap Screw" size "M3" standard "Ansi Metric M Profile"
sketch "Sketch20" plane through (7, -62.125, 16.25) normal (0, -1, 0) x (1, 0, 0)
  line L0 (74.272792, -11.706894) -> (58.111098, -11.706894) construction
  line L1 (58.111098, -11.706894) -> (58.111098, -3.568299) construction
  line L2 (58.111098, -3.568299) -> (74.272792, -3.568299) construction
  line L3 (74.272792, -3.568299) -> (74.272792, -11.706894) construction
  line L4 (74.249692, -11.568299) -> (71.662589, -11.568299)
  line L5 (71.662589, -11.568299) -> (69.853157, -5.808915)
  line L6 (69.853157, -5.808915) -> (68.082224, -11.568299)
  line L7 (68.082224, -11.568299) -> (65.572118, -11.568299)
  line L8 (65.572118, -11.568299) -> (68.544206, -3.568299)
  line L9 (68.544206, -3.568299) -> (71.223706, -3.568299)
  line L10 (71.223706, -3.568299) -> (74.249692, -11.568299)
  line L11 (58.611579, -3.568299) -> (65.279529, -3.568299)
  spline S0 degree 2 poles (65.279529, -3.568299) (65.164033, -4.553862) (64.001377, -6.293997) (62.399837, -7.479752) knots 0 0 0 1 2 2 2
  spline S1 degree 2 poles (62.399837, -7.479752) (61.429673, -8.203525) (60.882993, -8.958097) (60.882993, -9.296884) knots 0 0 0 1 2 2 2
  spline S2 degree 2 poles (60.882993, -9.296884) (60.882993, -9.66647) (61.421973, -10.182351) (61.830058, -10.182351) knots 0 0 0 1 2 2 2
  spline S3 degree 2 poles (61.830058, -10.182351) (62.261242, -10.182351) (62.800222, -9.651071) (62.892618, -8.973496) knots 0 0 0 1 2 2 2
  line L12 (62.892618, -8.973496) -> (65.117835, -9.15059)
  spline S4 degree 2 poles (65.117835, -9.15059) (64.98694, -10.089954) (64.286266, -11.144815) (63.015813, -11.706894) (61.891656, -11.706894) knots 0 0 0 1 2 3 3 3
  spline S5 degree 2 poles (61.891656, -11.706894) (60.7213, -11.706894) (59.412349, -11.167914) (58.665477, -10.066855) (58.665477, -9.373881) knots 0 0 0 1 2 3 3 3
  spline S6 degree 2 poles (58.665477, -9.373881) (58.665477, -8.642409) (59.520145, -7.310359) (60.652002, -6.509589) knots 0 0 0 1 2 2 2
  spline S7 degree 2 poles (60.652002, -6.509589) (61.321877, -6.047606) (61.77616, -5.67802) (62.084148, -5.377731) knots 0 0 0 1 2 2 2
  line L13 (62.084148, -5.377731) -> (58.611579, -5.377731)
  line L14 (58.611579, -5.377731) -> (58.611579, -3.568299)
  point P0 (-7, -16.25)
  constraints: 2 other
extrude "Extrusion16" cut sketch "Sketch20" against normal blind 0.5
body "Solid1"
